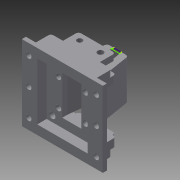
# Autodesk Inventor part: kraken_mount2
Saved by Autodesk Inventor 2014 (Build 180170000, 170)
## iProperties
Created: 2014-01-02
Part Number: kraken_mount2
Material: Generic
Document SubType Name: Modeling
Designer: stephen
Density: 1 g/cm^3
Appearance: Default
Author: stephen
Autodesk Inventor part; units mm, degrees
ref_plane "YZ Plane" through (0, 0, 0) normal (1, 0, 0) x (0, 1, 0)
ref_plane "XZ Plane" through (0, 0, 0) normal (0, 1, 0) x (-1, 0, 0)
sketch "Sketch1" plane through (0, 0, 0) normal (0, 1, 0) x (-1, 0, 0)
  line L0 (0, 0) -> (35.3, 0)
  line L1 (35.3, 0) -> (35.3, 40.3)
  line L2 (35.3, 40.3) -> (0, 40.3)
  line L3 (0, 40.3) -> (0, 0)
  line L4 (40.3, 45.3) -> (40.3, -5)
  line L5 (40.3, -5) -> (-5, -5)
  line L6 (-5, -5) -> (-5, 45.3)
  line L7 (-5, 45.3) -> (40.3, 45.3)
  dimension "d0" = 35.3
  dimension "d1" = 40.3
  dimension "d2" = 5
  constraints: 16 end point, 4 parallel, 2 perpendicular, 1 horizontal, 3 other
  measures "d0" distance of L2.end L1.end
  measures "d1" distance of L1.end L0.end
  measures "d2" distance between parallel lines of L6 L3
extrude "Extrusion1" add sketch "Sketch1" along normal blind 8
sketch "Sketch2" plane through (0, 8, 0) normal (0, 1, 0) x (1, 0, 0)
  line L0 (0, 0) -> (0, -40.3) projected
  line L1 (0, -40.3) -> (-35.3, -40.3) projected
  line L2 (-35.3, -40.3) -> (-35.3, 0) projected
  line L3 (-35.3, 0) -> (0, 0) projected
  line L4 (-32.15, -5.85) -> (-32.15, -35.15)
  line L5 (-29.8, -37.5) -> (-5.5, -37.5)
  line L6 (-3.15, -35.15) -> (-3.15, -5.85)
  circle A0 centre (-32.15, -3.5) radius 2.35
  circle A1 centre (-3.15, -3.5) radius 2.35
  circle A2 centre (-3.15, -37.5) radius 2.35
  circle A3 centre (-32.15, -37.5) radius 2.35
  line L7 (-5.5659, -5.5659) -> (-5.5659, -34.7341)
  line L8 (-5.5659, -34.7341) -> (-29.7341, -34.7341)
  line L9 (-29.7341, -34.7341) -> (-29.7341, -5.5659)
  line L10 (-29.7341, -5.5659) -> (-5.5659, -5.5659)
  line L11 (-5.5, -3.5) -> (-5.5659, -3.5)
  line L12 (-29.7341, -3.5) -> (-29.8, -3.5)
  dimension "d6" = 4.7
  dimension "d7" = 4.7
  dimension "d8" = 4.7
  dimension "d9" = 4.7
  dimension "d17" = 5.5659
  constraints: 18 end point, 8 point on circle, 4 centre point, 2 point on line, 3 other
  measures "d6" diameter of A0
  measures "d7" diameter of A1
  measures "d8" diameter of A2
  measures "d9" diameter of A3
  measures "d17" distance between parallel lines of L2 L9
extrude "Extrusion2" add sketch "Sketch2" against normal blind 4
sketch "Sketch3" plane through (0, 0, 0) normal (0, -1, 0) x (1, 0, 0)
  line L0 (-40.3, 45.3) -> (-40.3, -5) projected
  line L1 (-40.3, -5) -> (5, -5) projected
  line L2 (4.73, -7.79) -> (-40.03, -7.79)
  line L3 (-40.03, 48.09) -> (4.73, 48.09)
  line L4 (83.85, 15.65) -> (86.85, 15.65)
  circle A0 centre (25.35, 55.15) radius 2.5
  arc A1 (-22.4416, -21.2786) -> (-24.3582, -19.85) centre (-24.3582, -21.85) ccw
  line L5 (66.85, 24.65) -> (63.85, 24.65)
  line L6 (86.85, 10.65) -> (83.85, 10.65)
  circle A2 centre (25.35, 41.15) radius 2.5
  arc A3 (32.35, 38.15) -> (37.35, 33.15) centre (37.35, 38.15) ccw
  line L7 (2.35, 5.15) -> (2.35, 35.15)
  arc A4 (50.35, 7.15) -> (50.5801, 7.1553) centre (50.35, 12.15) ccw
  line L8 (-37.65, 35.15) -> (-37.65, 5.15)
  arc A5 (48.35, 26.15) -> (48.35, 30.15) centre (48.35, 28.15) ccw
  arc A6 (-22.4416, -21.2786) -> (-12.8584, -21.2786) centre (-17.65, -19.85) ccw
  line L9 (83.85, 43.65) -> (86.85, 43.65)
  line L10 (77.85, 41.65) -> (77.85, 38.15)
  arc A7 (86.85, 38.65) -> (86.85, 43.65) centre (86.85, 41.15) ccw
  line L11 (72.85, 33.15) -> (50.5801, 33.15)
  arc A8 (66.85, 24.65) -> (66.85, 29.65) centre (66.85, 27.15) ccw
  circle A9 centre (-42.65, 40.15) radius 2.1
  circle A10 centre (25.35, -14.85) radius 2.5
  arc A11 (83.85, 15.65) -> (83.85, 10.65) centre (83.85, 13.15) ccw
  line L12 (50.5801, 7.15) -> (72.85, 7.15)
  arc A12 (87.85, -6.35) -> (92.85, -1.35) centre (87.85, -1.35) ccw
  circle A13 centre (7.35, 40.15) radius 2.1
  line L13 (-47.65, 0.15) -> (-47.65, 40.15)
  arc A14 (92.85, 41.65) -> (87.85, 46.65) centre (87.85, 41.65) ccw
  arc A15 (66.85, 10.65) -> (66.85, 15.65) centre (66.85, 13.15) ccw
  line L14 (83.85, 29.65) -> (86.85, 29.65)
  line L15 (66.85, 10.65) -> (63.85, 10.65)
  arc A16 (-12.8584, 61.5786) -> (-10.9418, 60.15) centre (-10.9418, 62.15) ccw
  line L16 (83.85, 1.65) -> (86.85, 1.65)
  arc A17 (63.85, 15.65) -> (63.85, 10.65) centre (63.85, 13.15) ccw
  line L17 (48.35, 14.15) -> (38.35, 14.15)
  line L18 (-10.9418, 60.15) -> (27.35, 60.15)
  circle A18 centre (7.35, 0.15) radius 2.1
  line L19 (86.85, -3.35) -> (83.85, -3.35)
  line L20 (92.85, -1.35) -> (92.85, 41.65)
  arc A19 (86.85, -3.35) -> (86.85, 1.65) centre (86.85, -0.85) ccw
  line L21 (38.35, 10.15) -> (48.35, 10.15)
  arc A20 (82.85, 46.65) -> (77.85, 41.65) centre (82.85, 41.65) ccw
  arc A21 (86.85, 24.65) -> (86.85, 29.65) centre (86.85, 27.15) ccw
  line L22 (27.35, -19.85) -> (-10.9418, -19.85)
  arc A22 (-27.65, 60.15) -> (-47.65, 40.15) centre (-27.65, 40.15) ccw
  arc A23 (-10.9418, -19.85) -> (-12.8584, -21.2786) centre (-10.9418, -21.85) ccw
  line L23 (87.85, 46.65) -> (82.85, 46.65)
  arc A24 (48.35, 10.15) -> (48.35, 14.15) centre (48.35, 12.15) ccw
  circle A25 centre (-17.65, -19.85) radius 2.6
  line L24 (32.35, -14.85) -> (32.35, 2.15)
  arc A26 (83.85, 1.65) -> (83.85, -3.35) centre (83.85, -0.85) ccw
  arc A27 (86.85, 10.65) -> (86.85, 15.65) centre (86.85, 13.15) ccw
  circle A28 centre (25.35, 27.15) radius 2.5
  arc A29 (37.35, 7.15) -> (32.35, 2.15) centre (37.35, 2.15) ccw
  circle A30 centre (25.35, -0.85) radius 2.5
  line L25 (-27.65, 60.15) -> (-24.3582, 60.15)
  line L26 (-24.3582, -19.85) -> (-27.65, -19.85)
  line L27 (38.35, 26.15) -> (48.35, 26.15)
  circle A31 centre (-37.65, -12.85) radius 1.75
  line L28 (50.5801, 33.15) -> (50.5801, 33.1447)
  arc A32 (-17.8261, 55.1531) -> (-18.8441, 55.2947) centre (-17.65, 60.15) ccw
  arc A33 (72.85, 33.15) -> (77.85, 38.15) centre (72.85, 38.15) ccw
  arc A34 (38.35, 14.15) -> (38.35, 10.15) centre (38.35, 12.15) ccw
  arc A35 (83.85, 43.65) -> (83.85, 38.65) centre (83.85, 41.15) ccw
  line L29 (82.85, -6.35) -> (87.85, -6.35)
  circle A36 centre (2.35, 53.15) radius 1.75
  arc A37 (2.35, 35.15) -> (-37.65, 35.15) centre (-17.65, 35.15) ccw
  arc A38 (50.5801, 33.1447) -> (50.35, 33.15) centre (50.35, 28.15) ccw
  arc A39 (63.85, 29.65) -> (63.85, 24.65) centre (63.85, 27.15) ccw
  circle A40 centre (25.35, 13.15) radius 2.5
  arc A41 (77.85, -1.35) -> (82.85, -6.35) centre (82.85, -1.35) ccw
  circle A42 centre (-42.65, 20.15) radius 2.1
  arc A43 (-24.3582, 60.15) -> (-22.4416, 61.5786) centre (-24.3582, 62.15) ccw
  arc A44 (38.35, 30.15) -> (38.35, 26.15) centre (38.35, 28.15) ccw
  arc A45 (83.85, 29.65) -> (83.85, 24.65) centre (83.85, 27.15) ccw
  line L30 (50.35, 33.15) -> (37.35, 33.15)
  line L31 (50.35, 7.15) -> (37.35, 7.15)
  arc A46 (27.35, -19.85) -> (32.35, -14.85) centre (27.35, -14.85) ccw
  line L32 (86.85, 24.65) -> (83.85, 24.65)
  line L33 (50.5801, 7.1553) -> (50.5801, 7.15)
  circle A47 centre (7.35, 20.15) radius 2.1
  arc A48 (-37.65, 5.15) -> (2.35, 5.15) centre (-17.65, 5.15) ccw
  line L34 (63.85, 29.65) -> (66.85, 29.65)
  line L35 (48.35, 30.15) -> (38.35, 30.15)
  line L36 (77.85, 2.15) -> (77.85, -1.35)
  circle A49 centre (-17.65, 60.15) radius 2.6
  circle A50 centre (48.35, 20.15) radius 1.25
  line L37 (63.85, 15.65) -> (66.85, 15.65)
  arc A51 (-47.65, 0.15) -> (-27.65, -19.85) centre (-27.65, 0.15) ccw
  circle A52 centre (2.35, -12.85) radius 1.75
  arc A53 (32.35, 55.15) -> (27.35, 60.15) centre (27.35, 55.15) ccw
  arc A54 (77.85, 2.15) -> (72.85, 7.15) centre (72.85, 2.15) ccw
  circle A55 centre (-37.65, 53.15) radius 1.75
  circle A56 centre (-42.65, 0.15) radius 2.1
  line L38 (32.35, 38.15) -> (32.35, 55.15)
  line L39 (86.85, 38.65) -> (83.85, 38.65)
  circle A57 centre (38.35, 20.15) radius 1.25
  line L40 (-40.03, 48.09) -> (-47.6486, 48.09)
  line L41 (-47.6486, 48.09) -> (-47.6486, -7.79)
  line L42 (-47.6486, -7.79) -> (-40.03, -7.79)
  line L43 (4.73, 48.09) -> (12.35, 48.09)
  line L44 (12.35, 48.09) -> (12.35, -7.79)
  line L45 (12.35, -7.79) -> (4.73, -7.79)
  circle A58 centre (7.35, 40.15) radius 2.1
  circle A59 centre (7.35, 20.15) radius 2.1
  circle A60 centre (7.35, 0.15) radius 2.1
  circle A61 centre (-42.65, 40.15) radius 2.1
  circle A62 centre (-42.65, 0.15) radius 2.1
  circle A63 centre (-42.65, 20.15) radius 2.1
  line L46 (-40.3, 45.3) -> (5, 45.3)
  line L47 (5, 45.3) -> (5, -5)
  line L48 (5, -5) -> (-40.3, -5)
  line L49 (-40.3, -5) -> (-40.3, 45.3)
  line L50 (-47.6486, 48.09) -> (12.35, 48.09)
  line L51 (12.35, 48.09) -> (12.35, -7.79)
  line L52 (12.35, -7.79) -> (-47.6486, -7.79)
  line L53 (-47.6486, -7.79) -> (-47.6486, 48.09)
  point P0 (6.3945, 46.914)
  dimension "d12" = 7.62
  constraints: 104 end point, 81 tangent, 76 point on circle, 64 centre point, 55 equal radius, 26 parallel, 11 perpendicular, 6 coincident, 4 horizontal, 1 collinear, 1 concentric
  measures "d12" distance of L45.start L45.end
extrude "Extrusion3" add sketch "Sketch3" along normal blind 3 contours L0 L1 A48 L2 L42 A51 L13 A22 L40 L3 A37 L46 | A37 L3 L46 | L1 A48 L2 | A37 L3 L43 L44 L45 L2 A48 L1 L47 L46 | A22 L41 L40 | L42 L41 A51
sketch "Sketch5" plane through (0, -3, 0) normal (0, -1, 0) x (1, 0, 0)
  line L0 (-40.3, 45.3) -> (5, 45.3) projected
  line L1 (5, 45.3) -> (5, -5) projected
  line L2 (5, -5) -> (-40.3, -5) projected
  line L3 (-40.3, -5) -> (-40.3, 45.3) projected
  line L4 (0, 0) -> (-35.3, 0)
  line L5 (-35.3, 0) -> (-35.3, 40.3)
  line L6 (-35.3, 40.3) -> (0, 40.3)
  line L7 (0, 40.3) -> (0, 0)
  dimension "d15" = 35.3
  dimension "d16" = 40.3
  constraints: 8 end point, 2 parallel, 1 horizontal, 1 perpendicular
  measures "d15" distance of L5.end L6.end
  measures "d16" distance of L4.end L5.end
extrude "Extrusion4" add sketch "Sketch5" against normal up to next
sketch "Sketch6" plane through (0, 0, 0) normal (0, 1, 0) x (1, 0, 0)
  line L0 (-40.3, 5) -> (5, 5) projected
  line L1 (-47.6486, 7.79) -> (12.35, 7.79) projected
  line L2 (5, 5) -> (5, 23.7794)
  line L3 (5, 5) -> (23.7794, 5) construction
  line L4 (-40.3, 5) -> (-40.3, 33.7756)
  line L5 (-40.3, 7.79) -> (5, 7.79)
  line L6 (-40.3, 5) -> (5, 5)
  point P0 (0, 0)
  dimension "d20" = 90
  constraints: 10 end point, 4 point on line, 2 perpendicular, 1 collinear, 1 horizontal
  measures "d20" angle of L3 L2
extrude "Extrusion5" add sketch "Sketch6" along normal up to surface (8 mm away)
sketch "Sketch7" plane through (0, 0, 0) normal (0, 1, 0) x (1, 0, 0)
  line L0 (5, -45.3) -> (-40.3, -45.3) projected
  line L1 (12.35, -48.09) -> (-47.6486, -48.09) projected
  line L2 (5, 7.79) -> (12.35, 7.79) projected
  line L3 (-40.3, -45.3) -> (-40.3, -52.0309)
  line L4 (5, -45.3) -> (5, -53.1235)
  line L5 (5, -48.09) -> (-40.3, -48.09)
  line L6 (-40.3, -45.3) -> (5, -45.3)
  point P0 (0, 0)
  constraints: 8 end point, 4 point on line, 1 collinear, 1 parallel, 1 perpendicular
extrude "Extrusion6" add sketch "Sketch7" along normal up to surface (8 mm away)
sketch "Sketch8" plane through (0, 8, 0) normal (0, 1, 0) x (1, 0, 0)
  line L0 (-40.3, 7.79) -> (-40.3, -48.09) projected
  line L1 (5, -48.09) -> (5, 7.79) projected
  line L2 (5, 7.79) -> (-40.3, 7.79) projected
  line L3 (-40.3, 3.35) -> (5, 3.35)
  line L4 (5, -43.3291) -> (-40.3, -43.3291)
  point P0 (0, 0)
  dimension "d25" = 4.44
  constraints: 4 end point, 4 point on line, 2 perpendicular
  measures "d25" distance between parallel lines of L2 L3
extrude "Extrusion7" add sketch "Sketch8" along normal blind 19 contours L2 L1 L3 L0
sketch "Sketch9" plane through (0, 8, 0) normal (0, 1, 0) x (1, 0, 0)
  line L0 (-40.3, 3.35) -> (-40.3, -48.09) projected
  line L1 (-40.3, -48.09) -> (5, -48.09) projected
  line L2 (5, -48.09) -> (5, 3.35) projected
  line L3 (-40.3, -43.65) -> (5, -43.65)
  point P0 (0, 0)
  dimension "d28" = 4.44
  constraints: 2 end point, 2 point on line, 1 perpendicular
  measures "d28" distance between parallel lines of L1 L3
extrude "Extrusion8" add sketch "Sketch9" along normal blind 19
sketch "Sketch10" plane through (0, 8, 0) normal (0, 1, 0) x (1, 0, 0)
  line L0 (5, -43.65) -> (5, 3.35) projected
  line L1 (5, 3.35) -> (-40.3, 3.35) projected
  line L2 (-40.3, 3.35) -> (-40.3, -43.65) projected
  line L3 (-29.7341, -5.5659) -> (-5.5659, -5.5659) projected
  line L4 (-29.7341, -34.7341) -> (-29.7341, -5.5659) projected
  circle A0 centre (-3.15, -3.5) radius 2.35 projected
  circle A1 centre (-32.15, -3.5) radius 2.35 projected
  arc A2 (0.8186, -3) -> (-6.5752, -5.5659) centre (-3.15, -3.5) ccw
  line L5 (0.8186, -3) -> (5, -3)
  arc A3 (-27.4814, -3) -> (-36.8085, -2.9131) centre (-32.15, -3.5) ccw
  arc A4 (-29.7341, -6.9252) -> (-28.503, -5.5659) centre (-32.15, -3.5) ccw
  line L6 (-40.3, -2.9131) -> (-36.8085, -2.9131)
  line L7 (-27.4814, -3) -> (-7.1186, -3)
  line L8 (-40.3, -2.9131) -> (-40.3, 3.35)
  line L9 (5, 3.35) -> (5, -3)
  line L10 (5, 3.35) -> (-40.3, 3.35)
  point P0 (0, 0)
  dimension "d33" = 8
  constraints: 12 end point, 7 point on circle, 5 point on line, 3 centre point, 3 collinear, 3 perpendicular, 2 coincident
  measures "d33" diameter of A2
extrude "Extrusion9" add sketch "Sketch10" along normal blind 6.274 contours L5 A2 L7 A3 L6 L2 L1 L0
sketch "Sketch11" plane through (0, 8, 0) normal (0, 1, 0) x (1, 0, 0)
  circle A0 centre (-3.15, -37.5) radius 2.35 projected
  circle A1 centre (-32.15, -37.5) radius 2.35 projected
  line L0 (-5.5659, -34.7341) -> (-29.7341, -34.7341) projected
  line L1 (-40.3, -2.9131) -> (-40.3, -43.65) projected
  line L2 (-40.3, -43.65) -> (5, -43.65) projected
  line L3 (5, -43.65) -> (5, -3) projected
  arc A2 (-36.1186, -38) -> (-28.1814, -38) centre (-32.15, -37.5) ccw
  arc A3 (-6.0396, -34.7341) -> (0.8186, -38) centre (-3.15, -37.5) ccw
  line L4 (0.8186, -38) -> (5, -38)
  line L5 (-40.3, -38) -> (-36.1186, -38)
  line L6 (-28.1814, -38) -> (-7.1186, -38)
  line L7 (-40.3, -38) -> (-40.3, -43.65)
  line L8 (-40.3, -43.65) -> (5, -43.65)
  line L9 (5, -38) -> (5, -43.65)
  line L10 (5, -43.65) -> (-40.3, -43.65)
  point P0 (0, 0)
  dimension "d37" = 8
  dimension "d38" = 8
  constraints: 14 end point, 5 point on circle, 4 perpendicular, 3 collinear, 3 point on line, 2 centre point, 2 coincident
  measures "d37" diameter of A2
  measures "d38" diameter of A3
extrude "Extrusion10" add sketch "Sketch11" along normal blind 6.274 contours L5 A2 L6 A3 L4 L3 L2 L1
sketch "Sketch12" plane through (12.35, 0, -7.79) normal (0, 0, -1) x (-1, 0, 0)
  line L0 (52.65, 0) -> (52.65, 27) projected
  line L1 (7.35, 27) -> (52.65, 27) projected
  line L2 (59.9986, 0) -> (59.9986, -3) projected
  line L3 (52.65, 14.6559) -> (44.6903, 14.6559)
  circle A0 centre (37.6995, 17.5722) radius 1.967
  circle A1 centre (22.3005, 17.5722) radius 1.967
  line L4 (27.8781, 10.4279) -> (122.5324, 10.4279)
  line L5 (24.2675, 17.5722) -> (35.7325, 17.5722)
  line L6 (82.6836, 13.3441) -> (74.9841, 13.3441)
  line L7 (31, 17.5722) -> (31, 14.6559)
  line L8 (74.9841, 13.3441) -> (77.9003, 13.3441) construction
  line L9 (30, 27) -> (30, 13.9681)
  line L10 (44.6903, 14.6559) -> (30, 14.6559)
  point P0 (12.35, 0)
  dimension "d41" = 90
  dimension "d67" = 7.6995
  constraints: 16 end point, 4 perpendicular, 3 point on line, 2 horizontal alignment, 1 horizontal, 1 midpoint, 1 parallel, 4 other
  measures "d41" angle of L7 L8
  measures "d67" distance from line of L9 point (37.699, 17.572)
extrude "Extrusion11" cut sketch "Sketch12" against normal through all contours A0
sketch "Sketch13" plane through (12.35, 0, -7.79) normal (0, 0, -1) x (-1, 0, 0)
  circle A0 centre (37.7, 17.5722) radius 2.2225
  circle A1 centre (22.3, 17.5722) radius 2.15
  line L0 (23.523, 17.5722) -> (36.477, 17.5722)
  line L1 (30, 17.5722) -> (30, 14.2772)
  line L2 (30, 27) -> (30, 13.5)
  point P0 (12.35, 0)
  point P1 (30, 14.2772)
  dimension "d66" = 7.7
  dimension "d68" = 7.7
  dimension "d69" = 4.445
  dimension "d70" = 4.3
  constraints: 6 end point, 2 centre point, 1 midpoint, 1 point on line
  measures "d66" distance from line of L2 A0.centre
  measures "d68" distance from line of A1.centre L2
  measures "d69" diameter of A0
  measures "d70" diameter of A1
extrude "Extrusion12" cut sketch "Sketch13" against normal through all contours A1
sketch "Sketch14" plane through (12.35, 0, -7.79) normal (0, 0, -1) x (-1, 0, 0)
  line L0 (52.65, 0) -> (52.65, 27) projected
  line L1 (7.35, 27) -> (52.65, 27) projected
  line L2 (7.35, 0) -> (7.35, 27) projected
  line L3 (7.35, 14.1501) -> (16.35, 14.1501)
  line L4 (16.35, 14.1501) -> (16.35, 22.6508)
  line L5 (16.35, 22.6508) -> (43.65, 22.6508)
  line L6 (43.65, 14.1501) -> (43.65, 22.6508)
  line L7 (16.35, 22.6508) -> (43.65, 22.6508)
  line L8 (43.65, 22.6508) -> (43.65, 14.1501)
  line L9 (16.35, 14.1501) -> (16.35, 22.6508)
  line L10 (7.35, 14.1501) -> (16.35, 14.1501)
  line L11 (43.65, 14.1501) -> (52.65, 14.1501)
  point P0 (12.35, 0)
  point P1 (16.35, 27)
  point P2 (43.65, 27)
  dimension "d46" = 9
  constraints: 18 end point, 5 perpendicular, 3 point on line, 1 horizontal, 1 parallel
  measures "d46" distance of L3.end L3.start
extrude "Extrusion13" cut sketch "Sketch14" against normal through all
sketch "Sketch15" plane through (12.35, 0, -7.79) normal (0, 0, -1) x (-1, 0, 0)
  line L0 (52.65, 0) -> (52.65, 14.1501) projected
  line L1 (43.65, 14.1501) -> (52.65, 14.1501)
  line L2 (52.65, 14.1501) -> (52.65, 11.1501)
  line L3 (52.65, 11.1501) -> (43.65, 11.1501)
  line L4 (43.65, 11.1501) -> (43.65, 14.1501)
  point P0 (12.35, 0)
  dimension "d52" = 3
  constraints: 8 end point, 2 parallel, 1 horizontal, 1 perpendicular, 1 point on line
  measures "d52" distance of L1.end L2.end
extrude "Extrusion14" cut sketch "Sketch15" against normal blind 4.774
sketch "Sketch16" plane through (12.35, 0, -7.79) normal (0, 0, -1) x (-1, 0, 0)
  line L0 (7.35, 14.1501) -> (16.35, 14.1501)
  line L1 (16.35, 14.1501) -> (16.35, 11.1501)
  line L2 (16.35, 11.1501) -> (7.35, 11.1501)
  line L3 (7.35, 11.1501) -> (7.35, 14.1501)
  point P0 (12.35, 0)
  dimension "d55" = 3
  constraints: 8 end point, 2 parallel, 1 horizontal, 1 perpendicular
  measures "d55" distance of L0.end L1.end
extrude "Extrusion15" cut sketch "Sketch16" against normal blind 4.774
sketch "Sketch17" plane through (5, 0, 48.09) normal (0, 0, 1) x (1, 0, 0)
  line L0 (-45.3, 14.1501) -> (-36.3, 14.1501)
  line L1 (-36.3, 14.1501) -> (-36.3, 11.1501)
  line L2 (-36.3, 11.1501) -> (-45.3, 11.1501)
  line L3 (-45.3, 11.1501) -> (-45.3, 14.1501)
  point P0 (-5, 0)
  dimension "d58" = 3
  constraints: 8 end point, 2 parallel, 1 horizontal, 1 perpendicular
  measures "d58" distance of L0.end L1.end
extrude "Extrusion16" cut sketch "Sketch17" against normal blind 4.774
sketch "Sketch18" plane through (5, 0, 48.09) normal (0, 0, 1) x (1, 0, 0)
  line L0 (0, 0) -> (0, 14.1501) projected
  line L1 (-9, 14.1501) -> (0, 14.1501)
  line L2 (0, 14.1501) -> (0, 11.1501)
  line L3 (0, 11.1501) -> (-9, 11.1501)
  line L4 (-9, 11.1501) -> (-9, 14.1501)
  point P0 (-5, 0)
  dimension "d61" = 3
  constraints: 8 end point, 2 parallel, 1 horizontal, 1 perpendicular, 1 point on line
  measures "d61" distance of L1.end L2.end
extrude "Extrusion17" cut sketch "Sketch18" against normal blind 4.774
fillet "Fillet4" radius 2 8 edges at (-31.3, 22.6508, -5.57) (-40.3, 11.1501, -5.403) (-40.3, 8, 20.4565) (-40.3, 14.1501, -0.0515) (-4, 22.6508, -5.57) (5, 11.1501, -5.403) (5, 14.1501, -0.008) (5, 8, 20.5)
fillet "Fillet5" radius 2 6 edges at (-40.3, 11.1501, 45.703) (-40.3, 14.1501, 40.658) (-31.3, 22.6508, 45.87) (5, 11.1501, 45.703) (5, 14.1501, 40.658) (-4, 22.6508, 45.87)
sketch "Sketch19" plane through (0, 8, 0) normal (0, 1, 0) x (1, 0, 0)
  line L0 (-29.7341, -34.7341) -> (-29.7341, -5.5659) projected
  line L1 (-29.7341, -34.7341) -> (-29.7341, -5.5659)
  line L2 (-29.7341, -5.5659) -> (-24.7341, -5.5659)
  line L3 (-24.7341, -5.5659) -> (-24.7341, -34.7341)
  line L4 (-24.7341, -34.7341) -> (-29.7341, -34.7341)
  point P0 (0, 0)
  dimension "d71" = 5
  constraints: 8 end point, 3 equal length, 1 perpendicular
  measures "d71" distance of L0.end L2.end
extrude "Extrusion18" add sketch "Sketch19" against normal blind 4
sketch "Sketch20" plane through (0, 8, 0) normal (0, 1, 0) x (1, 0, 0)
  line L0 (-5.5659, -5.5659) -> (-5.5659, -34.7341) projected
  line L1 (-5.5659, -34.7341) -> (-5.5659, -5.5659)
  line L2 (-5.5659, -5.5659) -> (-10.5659, -5.5659)
  line L3 (-10.5659, -5.5659) -> (-10.5659, -34.7341)
  line L4 (-10.5659, -34.7341) -> (-5.5659, -34.7341)
  point P0 (0, 0)
  dimension "d74" = 5
  constraints: 8 end point, 3 equal length, 1 perpendicular
  measures "d74" distance of L2.end L0.start
extrude "Extrusion19" add sketch "Sketch20" against normal blind 4
sketch "Sketch21" plane through (0, 4, 0) normal (0, -1, 0) x (1, 0, 0)
  circle A0 centre (-32.15, 37.5) radius 2.35 projected
  circle A1 centre (-3.15, 37.5) radius 2.35 projected
  circle A2 centre (-3.15, 3.5) radius 2.35 projected
  circle A3 centre (-32.15, 3.5) radius 2.35 projected
  circle A4 centre (-27.65, 30.5) radius 2.075
  circle A5 centre (-27.65, 10.5) radius 2.075
  circle A6 centre (-7.65, 10.5) radius 2.075
  circle A7 centre (-7.65, 30.5) radius 2.075
  dimension "d77" = 4.15
  dimension "d78" = 4.5
  dimension "d79" = 7
  dimension "d94" = 4.15
  dimension "d95" = 4.15
  dimension "d96" = 4.15
  dimension "d97" = 4.5
  dimension "d98" = 7
  dimension "d99" = 7
  dimension "d100" = 4.5
  dimension "d101" = 7
  dimension "d102" = 4.5
  constraints: 4 centre point
  measures "d77" diameter of A4
  measures "d78" horizontal distance of A0.centre A4.centre
  measures "d79" vertical distance of A0.centre A4.centre
  measures "d94" diameter of A5
  measures "d95" diameter of A6
  measures "d96" diameter of A7
  measures "d97" horizontal distance of A5.centre A3.centre
  measures "d98" vertical distance of A5.centre A3.centre
  measures "d99" vertical distance of A2.centre A6.centre
  measures "d100" horizontal distance of A6.centre A2.centre
  measures "d101" vertical distance of A1.centre A7.centre
  measures "d102" horizontal distance of A7.centre A1.centre
ref_plane "Work Plane1" through (0, 41, 0) normal (0, 1, 0) x (1, 0, 0)
sketch "Sketch23" plane through (0, 8, 0) normal (0, 1, 0) x (1, 0, 0)
  line L0 (-24.7341, -34.7341) -> (-24.7341, -5.5659) projected
  line L1 (-24.7341, -34.7341) -> (-24.7341, -5.5659)
  line L2 (-24.7341, -5.5659) -> (-29.7341, -5.5659)
  line L3 (-29.7341, -5.5659) -> (-29.7341, -34.7341)
  line L4 (-29.7341, -34.7341) -> (-24.7341, -34.7341)
  line L5 (-7.1186, -3) -> (-27.4814, -3) projected
  line L6 (-10.5659, -34.7341) -> (-10.5659, -5.5659)
  line L7 (-10.5659, -5.5659) -> (-5.5659, -5.5659)
  line L8 (-5.5659, -5.5659) -> (-5.5659, -34.7341)
  line L9 (-5.5659, -34.7341) -> (-10.5659, -34.7341)
  point P0 (0, 0)
  dimension "d93" = 5
  dimension "d105" = 5
  constraints: 16 end point, 5 equal length, 3 perpendicular
  measures "d93" distance of L2.end L0.end
  measures "d105" distance of L6.end L7.end
sketch3d "3D Sketch2"
sketch "Sketch30" plane through (0, 8, 0) normal (0, 1, 0) x (1, 0, 0)
  line L0 (-24.7341, -34.7341) -> (-24.7341, -5.5659) projected
  line L1 (-28.1814, -38) -> (-7.1186, -38) projected
  line L2 (-24.7341, -5.5659) -> (-24.7341, -34.7341)
  line L3 (-24.7341, -34.7341) -> (-29.7341, -34.7341)
  line L4 (-29.7341, -34.7341) -> (-29.7341, -5.5659)
  line L5 (-29.7341, -5.5659) -> (-24.7341, -5.5659)
  point P0 (0, 0)
  dimension "d125" = 5
  constraints: 8 end point, 2 parallel, 2 perpendicular
  measures "d125" distance of L0.start L3.end
sketch3d "3D Sketch8"
  line L0 (-27.65, 4, 10.5) -> (-22.3342, 41, 11.557)
sweep "Sweep6" add profiles "Sketch30" path "3D Sketch8"
sketch3d "3D Sketch10"
  line L0 (-7.65, 4, 10.5) -> (-12.9154, 41, 11.557)
sweep "Sweep7" add profiles "Sketch23" path "3D Sketch10" contours L6 L7 L8 L9
sketch3d "3D Sketch11"
  line L0 (-7.65, 4, 30.5) -> (-12.9154, 41, 27.5403)
sweep "Sweep8" cut profiles "Sketch21" path "3D Sketch11" contours A7
sketch "Sketch32" plane through (0, 4, 0) normal (0, -1, 0) x (1, 0, 0)
  circle A0 centre (-3.15, 3.5) radius 2.35 projected
  circle A1 centre (-7.65, 10.5) radius 2.075
  point P0 (-4.0074, 5.6187)
  point P1 (-4.3697, 5.4516)
  dimension "d132" = 4.15
  dimension "d133" = 7
  dimension "d134" = 4.5
  constraints: 1 centre point, 1 other
  measures "d132" diameter of A1
  measures "d133" vertical distance of point (-3.15, 3.5) A1.centre
  measures "d134" horizontal distance of A1.centre point (-3.15, 3.5)
sketch3d "3D Sketch12"
  line L0 (-7.65, 4, 10.5) -> (-12.9154, 41, 11.557)
sweep "Sweep9" cut profiles "Sketch32" path "3D Sketch12" contours A1
sketch "Sketch33" plane through (0, 4, 0) normal (0, -1, 0) x (1, 0, 0)
  circle A0 centre (-32.15, 37.5) radius 2.35 projected
  circle A1 centre (-27.65, 30.5) radius 2.075
  dimension "d136" = 7
  dimension "d137" = 4.5
  constraints: 1 centre point
  measures "d136" vertical distance of A0.centre A1.centre
  measures "d137" horizontal distance of A1.centre A0.centre
sketch3d "3D Sketch13"
  line L0 (-27.55, 4, 30.3) -> (-22.3342, 41, 27.5403)
sweep "Sweep10" cut profiles "Sketch33" path "3D Sketch13" contours A1
sketch "Sketch34" plane through (0, 4, 0) normal (0, -1, 0) x (1, 0, 0)
  circle A0 centre (-27.55, 10.5) radius 2.075
  constraints: 1 centre point
sketch3d "3D Sketch14"
  line L0 (-27.65, 4, 10.5) -> (-22.3342, 41, 11.557)
sweep "Sweep11" cut profiles "Sketch34" path "3D Sketch14"
sketch "Sketch36" plane through (0, 41, 0) normal (0, 1, 0) x (1, 0, 0)
  line L0 (-27.6418, -4.2602) -> (-7.6287, -4.2602)
  line L1 (-7.6287, -4.2602) -> (-7.6287, -38.3418)
  line L2 (-7.6287, -38.3418) -> (-27.6418, -38.3418)
  line L3 (-27.6418, -38.3418) -> (-27.6418, -4.2602)
  point P0 (0, 0)
  constraints: 8 end point, 2 parallel, 1 horizontal, 1 perpendicular
extrude "Extrusion24" cut sketch "Sketch36" against normal blind 3
sketch "Sketch37" plane through (0, -3, 0) normal (0, -1, 0) x (1, 0, 0)
  line L0 (0, 40.3) -> (0, 0) projected
  line L1 (0, 0) -> (-35.3, 0) projected
  line L2 (-35.3, 0) -> (-35.3, 40.3) projected
  line L3 (-35.3, 40.3) -> (0, 40.3) projected
  line L4 (1, 41.3) -> (1, -1)
  line L5 (1, -1) -> (-36.3, -1)
  line L6 (-36.3, -1) -> (-36.3, 41.3)
  line L7 (-36.3, 41.3) -> (1, 41.3)
  dimension "d142" = 1
  constraints: 8 end point, 3 other
  measures "d142" distance between parallel lines of L7 L3
extrude "Extrusion25" cut sketch "Sketch37" against normal blind 7
fillet "Fillet8" radius 2 2 edges at (-9.8351, 38, 21.007) (-25.424, 38, 21.007)
sketch3d "3D Sketch15"
body "Solid1"
